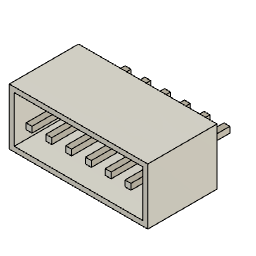
caja_EL6050 (Autodesk Fusion 360 archive; units mm, degrees)
design "JST6PIN2MM"
Autodesk Fusion 360 part; units mm, degrees
sketch "Sketch1" plane through (0, 0, 0) normal (0, 1, 0) x (1, 0, 0)
  line L0 (0, 0) -> (14, 0)
  line L1 (14, 0) -> (14, -5.7)
  line L2 (14, -5.7) -> (0, -5.7)
  line L3 (0, -5.7) -> (0, 0)
  line L4 (14, -2.85) -> (0, -2.85) construction
  line L5 (7, -5.7) -> (7, 0) construction
  line L6 (5.7, -3.15) -> (6.3, -3.15)
  line L7 (6.3, -3.15) -> (6.3, -2.55)
  line L8 (6.3, -2.55) -> (5.7, -2.55)
  line L9 (5.7, -2.55) -> (5.7, -3.15)
  line L10 (4.3, -2.55) -> (3.7, -2.55)
  line L11 (3.7, -3.15) -> (4.3, -3.15)
  line L12 (3.7, -2.55) -> (3.7, -3.15)
  line L13 (4.3, -3.15) -> (4.3, -2.55)
  line L14 (2.3, -2.55) -> (1.7, -2.55)
  line L15 (1.7, -3.15) -> (2.3, -3.15)
  line L16 (1.7, -2.55) -> (1.7, -3.15)
  line L17 (2.3, -3.15) -> (2.3, -2.55)
  line L18 (8.3, -2.55) -> (7.7, -2.55)
  line L19 (7.7, -3.15) -> (8.3, -3.15)
  line L20 (7.7, -2.55) -> (7.7, -3.15)
  line L21 (8.3, -3.15) -> (8.3, -2.55)
  line L22 (6.3, -2.55) -> (7.7, -3.15) construction
  line L23 (6.3, -3.15) -> (7.7, -2.55) construction
  line L24 (10.3, -3.15) -> (10.3, -2.55)
  line L25 (10.3, -2.55) -> (9.7, -2.55)
  line L26 (9.7, -3.15) -> (10.3, -3.15)
  line L27 (9.7, -2.55) -> (9.7, -3.15)
  line L28 (11.7, -3.15) -> (12.3, -3.15)
  line L29 (12.3, -2.55) -> (11.7, -2.55)
  line L30 (11.7, -2.55) -> (11.7, -3.15)
  line L31 (12.3, -3.15) -> (12.3, -2.55)
  line L32 (0.5, -0.5) -> (13.5, -0.5)
  line L33 (13.5, -0.5) -> (13.5, -5.2)
  line L34 (13.5, -5.2) -> (0.5, -5.2)
  line L35 (0.5, -5.2) -> (0.5, -0.5)
  dimension "d1" = 14
  dimension "d2" = 5.7
  dimension "d3" = 0.6
  dimension "d4" = 0.6
  dimension "d6" = 0.6
  dimension "d7" = 0.6
  dimension "d8" = 0.6
  dimension "d9" = 0.6
  dimension "d10" = 0.6
  dimension "d11" = 0.6
  dimension "d12" = 2
  dimension "d13" = 2
  dimension "d15" = 0.3
  dimension "d16" = 2
  dimension "d17" = 0.6
  dimension "d18" = 0.6
  dimension "d19" = 0.6
  dimension "d20" = 0.6
  dimension "d23" = 0.5
  constraint horizontal L0
  constraint vertical L1
  constraint horizontal L2
  constraint vertical L3
  constraint coincident L0.start L3.end
  constraint midpoint L1 L4.start
  constraint midpoint L3 L4.end
  constraint midpoint L2 L5.start
  constraint midpoint L0 L5.end
  constraint horizontal L6
  constraint vertical L7
  constraint horizontal L8
  constraint vertical L9
  constraint horizontal L11
  constraint vertical L13
  constraint horizontal L10
  constraint vertical L12
  constraint horizontal L15
  constraint vertical L17
  constraint horizontal L14
  constraint vertical L16
  constraint horizontal L19
  constraint vertical L21
  constraint horizontal L18
  constraint vertical L20
  constraint collinear L6 L11
  constraint collinear L11 L15
  constraint collinear L6 L19
  constraint midpoint L5 L22
  constraint horizontal L26
  constraint vertical L24
  constraint horizontal L25
  constraint vertical L27
  constraint horizontal L28
  constraint vertical L31
  constraint horizontal L29
  constraint vertical L30
  measures "d1" distance of L0.start L0.end
  measures "d2" distance of L0.start L2.end
  measures "d3" distance of L6.start L6.end
  measures "d4" distance of L6.start L8.end
  measures "d6" distance of L11.start L11.end
  measures "d7" distance of L11.start L10.end
  measures "d8" distance of L15.start L15.end
  measures "d9" distance of L15.start L14.end
  measures "d10" distance of L19.start L19.end
  measures "d11" distance of L19.start L18.end
  measures "d12" distance of L9 L12
  measures "d13" distance of L12 L16
  measures "d15" distance of L4 L6
  measures "d16" distance of L9 L20
  measures "d17" distance of L26.start L24.start
  measures "d18" distance of L26.start L25.end
  measures "d19" distance of L28.start L28.end
  measures "d20" distance of L28.start L29.end
extrude "Extrude1" add sketch "Sketch1" along normal blind 7 contours L0 L1 L2 L3 | L6 L7 L8 L9 | L10 L11 L12 L13 | L14 L15 L16 L17 | L18 L19 L20 L21 | L24 L25 L26 L27 | L28 L29 L30 L31 | L32 L33 L34 L35 makes body 1
extrude "Extrude2" cut sketch "Sketch1" along normal blind 6.5 contours L6 L7 L8 L9 | L10 L11 L12 L13 | L14 L15 L16 L17 | L18 L19 L20 L21 | L24 L25 L26 L27 | L28 L29 L30 L31 | L32 L33 L34 L35 bodies 1
extrude "Extrude3" add sketch "Sketch1" along normal blind 10 separate body contours L6 L7 L8 L9 | L10 L11 L12 L13 | L14 L15 L16 L17 | L18 L19 L20 L21 | L24 L25 L26 L27 | L28 L29 L30 L31 makes body 2 at (8.3, 6.6667, 2.95) makes body 3 at (2.3, 6.6667, 2.95) makes body 4 at (10.3, 6.6667, 2.95) makes body 5 at (6.3, 6.6667, 2.95) makes body 6 at (4.1, 6.6667, 2.55) makes body 7 at (11.7, 6.6667, 2.75)

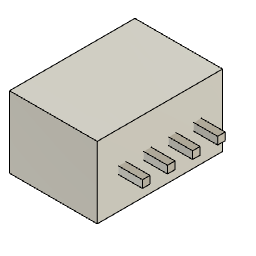
design "JST4PIN2MM"
Autodesk Fusion 360 part; units mm, degrees
sketch "Sketch2" plane through (0, 0, 0) normal (0, 0, 1) x (1, 0, 0)
  line L0 (0, 0) -> (7, 0)
  line L1 (7, 0) -> (7, 10)
  line L2 (7, 10) -> (0, 10)
  line L3 (0, 10) -> (0, 0)
  dimension "d1" = 7
  dimension "d2" = 10
  constraint horizontal L0
  constraint vertical L1
  constraint vertical L3
  constraint coincident L0.start L3.end
  measures "d1" distance of L0.start L0.end
  measures "d2" distance of L0.start L2.end
extrude "Extrude1" add sketch "Sketch2" along normal blind 5.7 makes body 1
sketch "Sketch4" plane through (0, 0, 0) normal (-1, 0, 0) x (0, -1, 0)
  line L0 (-10, 0) -> (0, 0)
  line L1 (0, 0) -> (0, 5.7)
  line L2 (0, 5.7) -> (-10, 5.7)
  line L3 (-10, 5.7) -> (-10, 0)
  line L4 (-10, 5.7) -> (0, 5.7)
  line L5 (0, 5.7) -> (0, 0)
  line L6 (0, 0) -> (-10, 0)
  line L7 (-10, 0) -> (-10, 5.7)
  line L8 (-0.5, 0.5) -> (-9.5, 0.5)
  line L9 (-9.5, 0.5) -> (-9.5, 5.2)
  line L10 (-9.5, 5.2) -> (-0.5, 5.2)
  line L11 (-0.5, 5.2) -> (-0.5, 0.5)
  line L12 (-10, 2.85) -> (0, 2.85) construction
  line L13 (-5, 5.7) -> (-5, 0) construction
  line L14 (-6, 5.2) -> (-6, 0.5) construction
  line L15 (-6.3, 3.15) -> (-5.7, 3.15)
  line L16 (-5.7, 3.15) -> (-5.7, 2.55)
  line L17 (-5.7, 2.55) -> (-6.3, 2.55)
  line L18 (-6.3, 2.55) -> (-6.3, 3.15)
  line L19 (-6.3, 3.15) -> (-5.7, 2.55) construction
  line L20 (-5.7, 3.15) -> (-6.3, 2.55) construction
  line L21 (-8.3, 2.55) -> (-8.3, 3.15)
  line L22 (-7.7, 2.55) -> (-8.3, 2.55)
  line L23 (-7.7, 3.15) -> (-7.7, 2.55)
  line L24 (-7.7, 3.15) -> (-8.3, 2.55) construction
  line L25 (-8.3, 3.15) -> (-7.7, 2.55) construction
  line L26 (-8.3, 3.15) -> (-7.7, 3.15)
  line L27 (-4.3, 2.55) -> (-4.3, 3.15)
  line L28 (-3.7, 2.55) -> (-4.3, 2.55)
  line L29 (-3.7, 3.15) -> (-3.7, 2.55)
  line L30 (-3.7, 3.15) -> (-4.3, 2.55) construction
  line L31 (-4.3, 3.15) -> (-3.7, 2.55) construction
  line L32 (-4.3, 3.15) -> (-3.7, 3.15)
  line L33 (-2.3, 2.55) -> (-2.3, 3.15)
  line L34 (-1.7, 2.55) -> (-2.3, 2.55)
  line L35 (-1.7, 3.15) -> (-1.7, 2.55)
  line L36 (-1.7, 3.15) -> (-2.3, 2.55) construction
  line L37 (-2.3, 3.15) -> (-1.7, 2.55) construction
  line L38 (-2.3, 3.15) -> (-1.7, 3.15)
  point P0 (-6, 2.85)
  point P1 (-8, 2.85)
  point P2 (-4, 2.85)
  point P3 (-2, 2.85)
  dimension "d23" = 0.5
  dimension "d24" = 1
  dimension "d25" = 0.6
  dimension "d26" = 0.6
  dimension "d27" = 0.6
  dimension "d28" = 0.6
  dimension "d29" = 0.6
  dimension "d30" = 0.6
  dimension "d31" = 0.6
  dimension "d32" = 0.6
  constraint horizontal L4
  constraint vertical L5
  constraint horizontal L6
  constraint vertical L7
  constraint coincident L0.end L1.start
  constraint coincident L2.end L3.start
  constraint midpoint L3 L12.start
  constraint midpoint L5 L12.end
  constraint midpoint L2 L13.start
  constraint midpoint L6 L13.end
  constraint coincident L10 L14.start
  constraint coincident L8 L14.end
  constraint perpendicular L8 L14
  constraint horizontal L15
  constraint perpendicular L15 L16
  constraint parallel L15 L17
  constraint parallel L16 L18
  constraint coincident L19 P0
  constraint coincident L20 P0
  constraint midpoint L14 P0
  constraint horizontal L26
  constraint perpendicular L23 L26
  constraint parallel L22 L26
  constraint parallel L21 L23
  constraint coincident P1 L25
  constraint coincident P1 L24
  constraint horizontal L32
  constraint perpendicular L29 L32
  constraint parallel L28 L32
  constraint parallel L27 L29
  constraint coincident P2 L31
  constraint coincident P2 L30
  constraint horizontal L38
  constraint perpendicular L35 L38
  constraint parallel L34 L38
  constraint parallel L33 L35
  constraint coincident P3 L37
  constraint coincident P3 L36
  measures "d24" distance of L13 L14
  measures "d25" distance of L16.end L17.end
  measures "d26" distance of L15.end L16.end
  measures "d27" distance of L22.start L21.start
  measures "d28" distance of L23.start L22.start
  measures "d29" distance of L28.start L27.start
  measures "d30" distance of L29.start L28.start
  measures "d31" distance of L34.start L33.start
  measures "d32" distance of L35.start L34.start
extrude "Extrude3" cut sketch "Sketch4" against normal blind 5.517 contours L8 L9 L10 L11 | L15 L16 L17 L18 | L21 L22 L23 L26 | L27 L28 L29 L32 | L33 L34 L35 L38 bodies 1
extrude "Extrude4" add sketch "Sketch4" against normal blind 8.906 separate body contours L15 L16 L17 L18 | L21 L22 L23 L26 | L27 L28 L29 L32 | L33 L34 L35 L38 makes body 2 at (2.9687, 5.7, 2.95) makes body 3 at (2.9687, 4.3, 2.75) makes body 4 at (2.9687, 8.3, 2.75) makes body 5 at (2.9687, 2.3, 2.75)
